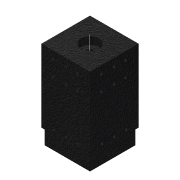
# Autodesk Inventor part: LASER_640nm
Saved by Autodesk Inventor 2019 (Build 230136000, 136)
## iProperties
Created: 2017-07-07
Part Number: LASER_640nm
Material: Generisch
Document SubType Name: Modeling
Designer: diederichbenedict
Density: 1 g/cm^3
Appearance: Schwarz - Guss
Author: diederichbenedict
Autodesk Inventor part; units mm, degrees
ref_plane "YZ Plane" through (0, 0, 0) normal (1, 0, 0) x (0, 1, 0)
ref_plane "XZ Plane" through (0, 0, 0) normal (0, 1, 0) x (-1, 0, 0)
ref_plane "XY Plane" through (0, 0, 0) normal (0, 0, 1) x (1, 0, 0)
sketch "Skizze1" plane through (0, 0, 0) normal (0, 0, 1) x (1, 0, 0)
  line L0 (-16, 16) -> (16, 16)
  line L1 (16, 16) -> (16, -16)
  line L2 (16, -16) -> (-16, -16)
  line L3 (-16, -16) -> (-16, 16)
  line L4 (-16, 16) -> (16, -16) construction
  line L5 (16, 16) -> (-16, -16) construction
  point P0 (0, 0)
  dimension "d0" = 32
  dimension "d1" = 32
  constraints: 12 end point, 2 midpoint, 2 parallel, 1 horizontal, 1 perpendicular
  measures "d0" distance of L1.end L2.end
  measures "d1" distance of L0.end L1.end
extrude "Extrusion1" add sketch "Skizze1" along normal blind 48
sketch "Skizze2" plane through (-16, 16, 0) normal (0, 1, 0) x (1, 0, 0)
  line L0 (0, 0) -> (32, 0) construction
  line L1 (0, 0) -> (0, -48) construction
  line L2 (32, -48) -> (0, -48) construction
  line L3 (32, 0) -> (32, -48) construction
  line L4 (5, -43) -> (5, -5)
  line L5 (5, -5) -> (27, -5)
  line L6 (27, -5) -> (27, -43)
  line L7 (27, -43) -> (5, -43)
  line L8 (32, -48) -> (0, -48) projected
  line L9 (16, -48) -> (16, 0)
  circle A0 centre (16, -5) radius 1
  circle A1 centre (8, -5) radius 1
  circle A2 centre (24, -5) radius 1
  circle A3 centre (16, -43) radius 1
  circle A4 centre (8.5, -43) radius 1
  circle A5 centre (24.5, -43) radius 1
  line L10 (27, -33) -> (5, -33)
  circle A6 centre (24.5, -33) radius 1.0474
  circle A7 centre (16, -33) radius 1
  circle A8 centre (8.5, -33) radius 1
  circle A9 centre (8, -3) radius 1
  circle A10 centre (16, -3) radius 1
  circle A11 centre (24, -3) radius 1
  dimension "d4" = 5
  dimension "d5" = 2
  dimension "d6" = 2
  dimension "d7" = 2
  dimension "d8" = 2
  dimension "d9" = 8
  dimension "d10" = 8
  dimension "d11" = 2
  dimension "d12" = 2
  dimension "d23" = 10
  dimension "d31" = 2
  dimension "d32" = 2
  dimension "d33" = 2
  dimension "d37" = 30
  dimension "d38" = 0
  dimension "d39" = 0
  constraints: 12 centre point, 12 end point, 11 point on line, 4 midpoint, 1 perpendicular, 1 vertical, 3 other
  measures "d4" distance between parallel lines of L1 L4
  measures "d5" diameter of A0
  measures "d6" diameter of A1
  measures "d7" diameter of A2
  measures "d8" diameter of A3
  measures "d9" distance of A1.centre A0.centre
  measures "d10" distance of A2.centre A0.centre
  measures "d11" diameter of A4
  measures "d12" diameter of A5
  measures "d23" distance between parallel lines of L10 L7
  measures "d31" diameter of A9
  measures "d32" diameter of A10
  measures "d33" diameter of A11
  measures "d37" vertical distance of A8.centre A9.centre
  measures "d38" vertical distance of A10.centre A9.centre
  measures "d39" vertical distance of A11.centre A10.centre
extrude "Extrusion2" cut sketch "Skizze2" against normal blind 8 contours A9 | A10 L9 | L9 A10 | A11 | A4 L7 | L7 A4 | A8 L10 | L10 A8 | A3 L9 L7 | L7 L9 A3 | A7 L9 L10 | L10 L9 A7 | L9 A3 L7 | L7 A3 L9 | L10 A7 L9 | L9 A7 L10 | A5 L7 | L7 A5 | A6 L10 | L10 A6
sketch "Skizze3" plane through (0, 0, 48) normal (0, 0, 1) x (1, 0, 0)
  circle A0 centre (0, 0) radius 2.5
  dimension "d15" = 5
  constraints: 1 centre point, 1 coincident
  measures "d15" diameter of A0
extrude "Extrusion3" cut sketch "Skizze3" against normal through all
sketch "Skizze4" plane through (0, 0, 48) normal (0, 0, 1) x (1, 0, 0)
  line L0 (-2.45, 0.55) -> (-42.45, 0.55) projected
  circle A0 centre (0, 0) radius 2.5 projected
  line L1 (16, 16) -> (-16, 16) projected
  line L2 (-16, 16) -> (-16, -16) projected
  line L3 (-16, -16) -> (16, -16) projected
  line L4 (16, -16) -> (16, 16) projected
  circle A1 centre (0, 0) radius 6
  dimension "d18" = 12
  constraints: 1 centre point, 1 coincident
  measures "d18" diameter of A1
extrude "Extrusion4" cut sketch "Skizze4" against normal blind 5 contours A1
sketch "Skizze5" plane through (0, 0, 0) normal (0, 0, -1) x (-1, 0, 0)
  line L0 (-15, -15) -> (15, -15)
  line L1 (15, -15) -> (15, 15)
  line L2 (15, 15) -> (-15, 15)
  line L3 (-15, 15) -> (-15, -15)
  circle A0 centre (0, 0) radius 2.5 projected
  line L4 (-15, -15) -> (15, 15) construction
  line L5 (15, -15) -> (-15, 15) construction
  dimension "d24" = 30
  dimension "d25" = 30
  constraints: 12 end point, 2 midpoint, 2 parallel, 1 horizontal, 1 perpendicular
  measures "d24" distance of L2.end L1.end
  measures "d25" distance of L1.end L0.end
extrude "Extrusion5" add sketch "Skizze5" along normal blind 10
pattern_circular "Runde Anordnung1" count 4 over 360 about axis through (0, 0, 48) along (0, 0, -1) of "Extrusion2"
